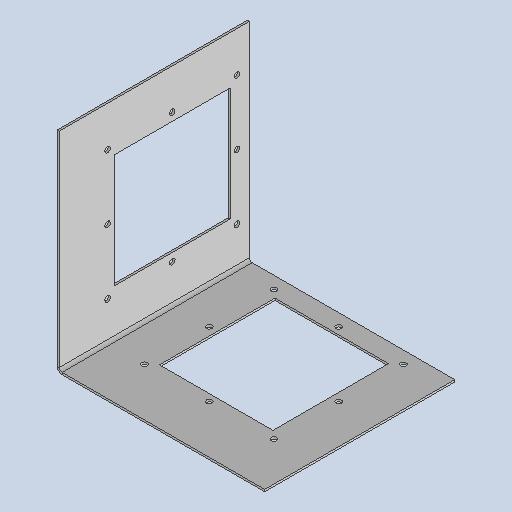
# Autodesk Inventor part: NDV-1101 Center wall 01
Saved by Autodesk Inventor 2026.2 (Build 302298000, 298)
## iProperties
Created: 2025-06-24
Part Number: NDV-1101 Center wall 01
Material: Stainless Steel
Document SubType Name: Sheet Metal
Designer: admin
Mass: 728.638 g
Surface Area: 958.262 cm^2
Volume: 91.0797 cm^3
Density: 8 g/cm^3
Flat Pattern Width: 40.2202 cm
Flat Pattern Length: 18.5 cm
Flat Pattern Area: 744.074 cm^2
Sheet Metal Rule: AISI304 2mm Die16
Sheet Metal Width: 402,202 mm
Sheet Metal Length: 185,000 mm
Sheet Metal Area: 74407,368 mm^2
Appearance: Default
Stock Number: Стенка центра
Author: user
Autodesk Inventor part; units mm, degrees
ref_plane "YZ Plane" through (0, 0, 0) normal (1, 0, 0) x (0, 1, 0)
ref_plane "XZ Plane" through (0, 0, 0) normal (0, 1, 0) x (-1, 0, 0)
sketch "Sketch1" plane through (0, 0, 0) normal (0, 0, 1) x (1, 0, 0)
  line L0 (-101, -92.5) -> (101, -92.5)
  line L1 (101, -92.5) -> (101, 92.5)
  line L2 (101, 92.5) -> (-101, 92.5)
  line L3 (-101, 92.5) -> (-101, -92.5)
  line L4 (-101, -92.5) -> (101, 92.5) construction
  line L5 (101, -92.5) -> (-101, 92.5) construction
  line L6 (55.25, 73.75) -> (-55.25, 73.75)
  line L7 (-55.25, 73.75) -> (-55.25, -38.75)
  line L8 (-55.25, -38.75) -> (55.25, -38.75)
  line L9 (55.25, -38.75) -> (55.25, 73.75)
  point P0 (0, 0)
  dimension "d154" = 202
  dimension "d155" = 185
  dimension "d185" = 110.5
  dimension "d186" = 112.5
  dimension "d187" = 45.75
  dimension "d188" = 45.75
  dimension "d190" = 18.75
  measures "d154" distance of L1.end L2.end
  measures "d155" distance of L0.end L1.end
  measures "d185" distance of L8.end L7.end
  measures "d186" distance of L7.end L6.end
  measures "d187" distance between parallel lines of L7 L3
  measures "d188" distance between parallel lines of L1 L9
  measures "d190" distance between parallel lines of L6 L2
extrude "Plate5" add sketch "Sketch1" along normal blind 2
sketch "Sketch7" plane through (-99, -92.5, 0) normal (-1, 0, 0) x (0, -1, 0)
  line L0 (-185, 0) -> (0, 0)
  line L1 (0, 0) -> (0, 204)
  line L2 (0, 204) -> (-185, 204)
  line L3 (-185, 204) -> (-185, 0)
  constraints: 6 end point, 1 horizontal, 1 perpendicular, 1 vertical
edge flange "Flange3" height 204 angle 90 thickness 2 bend radius 2.75 thickness toward (-1, 0, 0) relief round relief width 2 relief depth 1 edges at (-101, 0, 2) wall of the first edge with corners at (-99, 92.5, 0) (-99, -92.5, 0) (-99, -92.5, 204) (-99, 92.5, 204)
bend "Bend3"
corner "Corner3"
derived "NDV-0010 Parameters 01.ipt"
sketch "sk_windowB" plane through (-101, -92.5, 204) normal (-1, 0, 0) x (0, 0, 1)
  line L0 (0, 185) -> (0, 0) projected
  line L1 (-199.25, 185) -> (0, 185) projected
  line L2 (-157.25, 53.75) -> (-157.25, 166.25)
  line L3 (-157.25, 166.25) -> (-46.75, 166.25)
  line L4 (-46.75, 166.25) -> (-46.75, 53.75)
  line L5 (-46.75, 53.75) -> (-157.25, 53.75)
  circle A0 centre (-165, 173) radius 2.75
  circle A1 centre (-39, 173) radius 2.75
  circle A2 centre (-39, 47) radius 2.75
  circle A3 centre (-165, 47) radius 2.75
  circle A4 centre (-102, 173) radius 2.75
  circle A5 centre (-102, 47) radius 2.75
  circle A6 centre (-165, 110) radius 2.75
  circle A7 centre (-39, 110) radius 2.75
  dimension "d222" = 46.75
  dimension "d223" = 18.75
  dimension "d224" = 110.5
  dimension "d225" = 112.5
  dimension "d226" = 5.5
  dimension "d227" = 7.75
  dimension "d228" = 6.75
  dimension "d229" = 5.5
  dimension "d230" = 7.75
  dimension "d231" = 6.75
  dimension "d232" = 5.5
  dimension "d233" = 7.75
  dimension "d234" = 6.75
  dimension "d235" = 5.5
  dimension "d236" = 7.75
  dimension "d237" = 6.75
  dimension "d238" = 5.5
  dimension "d239" = 55.25
  dimension "d240" = 6.75
  dimension "d241" = 5.5
  dimension "d242" = 55.25
  dimension "d243" = 6.75
  dimension "d244" = 5.5
  dimension "d245" = 7.75
  dimension "d246" = 56.25
  dimension "d247" = 5.5
  dimension "d248" = 7.75
  dimension "d249" = 56.25
  constraints: 8 centre point, 8 end point, 3 perpendicular, 1 parallel
  measures "d222" distance from line of L0 L3.end
  measures "d223" distance from line of L1 L2.end
  measures "d224" distance from line of L4 L2.start
  measures "d225" distance from line of L3 L4.end
  measures "d226" diameter of A0
  measures "d227" distance from line of L2 A0.centre
  measures "d228" distance from line of L3 A0.centre
  measures "d229" diameter of A1
  measures "d230" distance from line of L4 A1.centre
  measures "d231" distance from line of L3 A1.centre
  measures "d232" diameter of A2
  measures "d233" distance from line of L4 A2.centre
  measures "d234" distance from line of L5 A2.centre
  measures "d235" diameter of A3
  measures "d236" distance from line of L2 A3.centre
  measures "d237" distance from line of L5 A3.centre
  measures "d238" diameter of A4
  measures "d239" distance from line of L2 A4.centre
  measures "d240" distance from line of L3 A4.centre
  measures "d241" diameter of A5
  measures "d242" distance from line of L2 A5.centre
  measures "d243" distance from line of L5 A5.centre
  measures "d244" diameter of A6
  measures "d245" distance from line of L2 A6.centre
  measures "d246" distance from line of L3 A6.centre
  measures "d247" diameter of A7
  measures "d248" distance from line of L4 A7.centre
  measures "d249" distance from line of L3 A7.centre
extrude "Cut_windowB" cut sketch "sk_windowB" against normal blind 2
sketch "sk_rivetsA" plane through (0, 0, 0) normal (0, 0, -1) x (-1, 0, 0)
  line L0 (55.25, -38.75) -> (-55.25, -38.75) projected
  line L1 (-55.25, -38.75) -> (-55.25, 73.75) projected
  line L2 (-55.25, 73.75) -> (55.25, 73.75) projected
  line L3 (55.25, 73.75) -> (55.25, -38.75) projected
  circle A0 centre (-63, 80.5) radius 2.75
  circle A1 centre (63, 80.5) radius 2.75
  circle A2 centre (63, -45.5) radius 2.75
  circle A3 centre (-63, -45.5) radius 2.75
  circle A4 centre (0, 80.5) radius 2.75
  circle A5 centre (0, -45.5) radius 2.75
  circle A6 centre (-63, 17.5) radius 2.75
  circle A7 centre (63, 17.5) radius 2.75
  dimension "d252" = 5.5
  dimension "d253" = 7.75
  dimension "d254" = 6.75
  dimension "d255" = 5.5
  dimension "d256" = 7.75
  dimension "d257" = 6.75
  dimension "d258" = 5.5
  dimension "d259" = 7.75
  dimension "d260" = 6.75
  dimension "d261" = 5.5
  dimension "d262" = 7.75
  dimension "d263" = 6.75
  dimension "d264" = 5.5
  dimension "d265" = 55.25
  dimension "d266" = 6.75
  dimension "d267" = 5.5
  dimension "d268" = 55.25
  dimension "d269" = 6.75
  dimension "d270" = 5.5
  dimension "d271" = 7.75
  dimension "d272" = 56.25
  dimension "d273" = 5.5
  dimension "d274" = 7.75
  dimension "d275" = 56.25
  constraints: 8 centre point
  measures "d252" diameter of A0
  measures "d253" distance from line of L1 A0.centre
  measures "d254" distance from line of L2 A0.centre
  measures "d255" diameter of A1
  measures "d256" distance from line of L3 A1.centre
  measures "d257" distance from line of L2 A1.centre
  measures "d258" diameter of A2
  measures "d259" distance from line of L3 A2.centre
  measures "d260" distance from line of L0 A2.centre
  measures "d261" diameter of A3
  measures "d262" distance from line of L1 A3.centre
  measures "d263" distance from line of L0 A3.centre
  measures "d264" diameter of A4
  measures "d265" distance from line of L1 A4.centre
  measures "d266" distance from line of L2 A4.centre
  measures "d267" diameter of A5
  measures "d268" distance from line of L1 A5.centre
  measures "d269" distance from line of L0 A5.centre
  measures "d270" diameter of A6
  measures "d271" distance from line of L1 A6.centre
  measures "d272" distance from line of L2 A6.centre
  measures "d273" diameter of A7
  measures "d274" distance from line of L3 A7.centre
  measures "d275" distance from line of L2 A7.centre
extrude "Cut_rivetsA" cut sketch "sk_rivetsA" against normal blind 2 contours A0 | A1 | A2 | A3 | A4 | A5 | A6 | A7
ref_plane "BoxCenter" through (0, 0, 102) normal (0, 0, 1) x (1, 0, 0)
body "Solid3"
